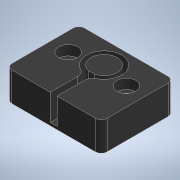
# Autodesk Inventor part: 19_Belt_holder
Saved by Autodesk Inventor 2022.2 (Build 262287010, 287A)
## iProperties
Created: 2022-04-30
Part Number: 19_Belt_holder
Material: PET-Kunststoff
Document SubType Name: Modeling
Designer: MXBD
Density: 1.541 g/cm^3
Appearance: Gummi - Schwarz
Author: MXBD
Autodesk Inventor part; units mm, degrees
ref_plane "YZ Plane" through (0, 0, 0) normal (1, 0, 0) x (0, 1, 0)
ref_plane "XZ Plane" through (0, 0, 0) normal (0, 1, 0) x (-1, 0, 0)
ref_plane "XY Plane" through (0, 0, 0) normal (0, 0, 1) x (1, 0, 0)
sketch "Skizze1" plane through (0, 0, 0) normal (0, 1, 0) x (-1, 0, 0)
  line L0 (-16.35, 12.5) -> (16.35, 12.5)
  line L1 (16.35, 12.5) -> (16.35, -12.5)
  line L2 (16.35, -12.5) -> (-16.35, -12.5)
  line L3 (-16.35, -12.5) -> (-16.35, 12.5)
  line L4 (-16.35, 12.5) -> (16.35, -12.5) construction
  line L5 (16.35, 12.5) -> (-16.35, -12.5) construction
  point P0 (0, 0)
  dimension "d0" = 32.7
  dimension "d1" = 25
  constraints: 12 end point, 2 midpoint, 2 parallel, 1 horizontal, 1 perpendicular
  measures "d0" distance of L1.end L2.end
  measures "d1" distance of L0.end L1.end
extrude "Extrusion1" add sketch "Skizze1" along normal blind 10
sketch "Skizze3" plane through (0, 10, 0) normal (0, 1, 0) x (1, 0, 0)
  line L0 (0, 17.5) -> (0, -17.5) projected
  line L1 (-16.35, -12.5) -> (16.35, -12.5) projected
  line L2 (-1.15, -12.5) -> (1.15, -12.5)
  line L3 (1.15, -12.5) -> (1.15, 0.5)
  line L4 (1.15, 0.5) -> (-1.15, 0.5)
  line L5 (-1.15, 0.5) -> (-1.15, -12.5)
  point P0 (0, 0)
  point P1 (1.15, -12.5)
  dimension "d11" = 2.3
  dimension "d12" = 13
  constraints: 8 end point, 2 parallel, 1 horizontal, 1 perpendicular, 1 point on line, 1 other
  measures "d11" distance between parallel lines of L3 L5
  measures "d12" distance between parallel lines of L1 L4
extrude "Extrusion2" cut sketch "Skizze3" against normal blind 9
sketch "Skizze4" plane through (0, 10, 0) normal (0, 1, 0) x (1, 0, 0)
  line L0 (-1.15, -12.5) -> (-1.15, 0.5) projected
  circle A0 centre (0, 4.8506) radius 4.5
  line L1 (0, 17.5) -> (0, -17.5) projected
  circle A1 centre (0, 4.8506) radius 6
  point P0 (0, 0)
  point P1 (-1.15, -1.0382)
  point P2 (0, 0.3506)
  point P3 (0, 10.8506)
  point P4 (0, 9.3506)
  point P5 (0, -1.1494)
  dimension "d16" = 9
  dimension "d17" = 1.5
  constraints: 1 centre point, 1 coincident, 1 point on line, 3 other
extrude "Extrusion3" cut sketch "Skizze4" against normal up to surface (9 mm away) contours A1 L1 A0 L0 | L0 A0 L1 A1 | A1 L1 A0
fillet "Rundung1" radius 3 2 edges at (-1.15, 5.5, 1.0382) (1.15, 5.5, 1.0382)
sketch "Skizze5" plane through (0, 10, 0) normal (0, 1, 0) x (1, 0, 0)
  line L0 (0, 17.5) -> (0, -17.5) projected
  line L1 (16.35, 12.5) -> (-16.35, 12.5) projected
  point P0 (0, 0)
  point P1 (-10, 2.5)
  point P2 (10, 2.5)
  dimension "d21" = 10
  dimension "d22" = 20
  constraints: 1 symmetric about line
  measures "d21" distance from line of point (-10, 2.5) L1
  measures "d22" distance of point (10, 2.5) point (-10, 2.5)
hole "Bohrung2" at (-10, 10, -2.5) at (10, 10, -2.5) direction (0, -1, 0) diameter 3.4 end through all counterbore diameter 6.5 counterbore depth 3.4 clearance for "Inbusschraube ISO 4762" size "M3" standard "ISO"
fillet "Rundung2" radius 2 4 edges at (16.35, 5, 12.5) (16.35, 5, -12.5) (-16.35, 5, -12.5) (-16.35, 5, 12.5)
